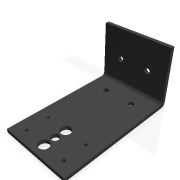
# Autodesk Inventor part: Part5
Saved by Autodesk Inventor 2019 (Build 230136000, 136)
## iProperties
Created: 2019-07-18
Part Number: Part5
Material: Generic
Document SubType Name: Modeling
Designer: romanp
Density: 1 g/cm^3
Appearance: Default
Author: romanp
Autodesk Inventor part; units mm, degrees
ref_plane "YZ Plane" through (0, 0, 0) normal (1, 0, 0) x (0, 1, 0)
ref_plane "XZ Plane" through (0, 0, 0) normal (0, 1, 0) x (-1, 0, 0)
ref_plane "XY Plane" through (0, 0, 0) normal (0, 0, 1) x (1, 0, 0)
sketch "Sketch1" plane through (0, 0, 0) normal (0, 0, 1) x (1, 0, 0)
  line L0 (0, 0) -> (0, 60)
  line L1 (0, 60) -> (70, 60)
  line L2 (70, 60) -> (70, 0)
  line L3 (70, 0) -> (0, 0)
  dimension "d0" = 60
  dimension "d1" = 70
  dimension "d2" = 60
  constraints: 8 end point, 2 perpendicular, 1 vertical
  measures "d0" distance of L0.start L0.end
  measures "d1" distance of L0.end L1.end
  measures "d2" distance of L1.end L2.end
extrude "Extrusion1" add sketch "Sketch1" along normal blind 4
sketch "Sketch2" plane through (0, 0, 4) normal (0, 0, 1) x (1, 0, 0)
  line L0 (0, 0) -> (70, 0) projected
  line L1 (70, 0) -> (70, 60) projected
  line L2 (0, 0) -> (70, 0)
  line L3 (70, 0) -> (70, 4)
  line L4 (70, 4) -> (0, 4)
  line L5 (0, 4) -> (0, 0)
  dimension "d5" = 4
  constraints: 8 end point, 2 parallel, 1 horizontal, 1 perpendicular, 1 point on line
  measures "d5" distance of L3.end L2.end
extrude "Extrusion2" add sketch "Sketch2" along normal blind 115
sketch "Sketch3" plane through (0, 0, 0) normal (0, 0, -1) x (-1, 0, 0)
  line L0 (-70, 60) -> (-70, 0) projected
  circle A0 centre (-50, 30) radius 3
  circle A1 centre (-20, 30) radius 3
  dimension "d15" = 6
  dimension "d16" = 6
  constraints: 2 centre point
  measures "d15" diameter of A0
  measures "d16" diameter of A1
extrude "Extrusion3" cut sketch "Sketch3" against normal blind 10
sketch "Sketch4" plane through (0, 0, 0) normal (0, -1, 0) x (1, 0, 0)
  line L0 (70, 0) -> (70, 119) projected
  line L1 (23, 0) -> (17, 0) projected
  line L2 (17, 0) -> (23, 0)
  circle A0 centre (50, 23) radius 3
  circle A1 centre (20, 23) radius 3
  dimension "d26" = 6
  dimension "d27" = 6
  constraints: 2 centre point, 2 end point, 1 collinear
  measures "d26" diameter of A0
  measures "d27" diameter of A1
extrude "Extrusion4" cut sketch "Sketch4" against normal blind 10
sketch "Sketch5" plane through (0, 0, 0) normal (0, -1, 0) x (1, 0, 0)
  line L0 (70, 4) -> (70, 119) projected
  circle A0 centre (50, 23) radius 3 projected
  circle A1 centre (35, 108.75) radius 5.25
  circle A2 centre (35, 86.75) radius 5.25
  circle A3 centre (35, 97.75) radius 4
  circle A4 centre (55.25, 86.75) radius 2
  circle A5 centre (55.25, 108.75) radius 2
  circle A6 centre (14.75, 86.75) radius 2
  circle A7 centre (14.75, 108.75) radius 2
  point P0 (0, 0)
  point P1 (20, 23)
  dimension "d36" = 8
  dimension "d41" = 4
  dimension "d42" = 4
  dimension "d43" = 4
  dimension "d44" = 4
  constraints: 7 centre point
  measures "d36" diameter of A3
  measures "d41" diameter of A4
  measures "d42" diameter of A5
  measures "d43" diameter of A6
  measures "d44" diameter of A7
extrude "Extrusion5" cut sketch "Sketch5" against normal blind 10 contours A1 | A2 | A3 | A4 | A5 | A6 | A7
sketch "Sketch6" plane through (70, 0, 0) normal (1, 0, 0) x (0, 0, -1)
  line L0 (0, 0) -> (-119, 0) projected
  line L1 (0, 4) -> (0, 4)
  line L2 (-4, 4) -> (-119, 4) projected
  line L3 (0, 60) -> (0, 0) projected
  line L4 (-4, 0) -> (-4, 0)
  arc A0 (-4, 0) -> (0, 4) centre (-4, 4) ccw
  line L5 (0, 4) -> (0, 0)
  line L6 (-4, 0) -> (0, 0)
  dimension "d47" = 4
  dimension "d48" = 4
  dimension "d49" = 4
  constraints: 8 end point, 4 tangent, 3 point on line, 2 collinear, 2 point on circle, 1 centre point, 1 perpendicular
  measures "d47" distance of L0.start L1.end
  measures "d48" distance of L0.start L4.end
  measures "d49" radius of A0
extrude "Extrusion6" cut sketch "Sketch6" against normal blind 100
sketch "Sketch7" plane through (70, 60, 4) normal (1, 0, 0) x (0, 0, -1)
  line L0 (0, -56) -> (0, 0) projected
  line L1 (0, -52) -> (0, -52)
  line L2 (-4, -56) -> (-4, -56)
  arc A0 (-4, -56) -> (0, -52) centre (-4, -52) ccw
  line L3 (0, -52) -> (0, -56)
  line L4 (0, -56) -> (-115, -56) projected
  line L5 (-4, -56) -> (0, -56)
  point P0 (4, -60)
  dimension "d52" = 4
  dimension "d53" = 4
  dimension "d54" = 4
  constraints: 8 end point, 4 tangent, 3 point on line, 2 collinear, 2 point on circle, 1 centre point, 1 horizontal
  measures "d52" distance of L0.start L1.end
  measures "d53" distance of L0.start L2.end
  measures "d54" radius of A0
extrude "Extrusion7" add sketch "Sketch7" against normal blind 70
sketch "Sketch8" plane through (0, 0, 119) normal (0, -1, 0) x (1, 0, 0)
  circle A0 centre (35, -10.25) radius 5.25 projected
  circle A1 centre (55.25, -32.25) radius 2 projected
  circle A2 centre (55.25, -32.25) radius 2
  circle A3 centre (55.25, -10.25) radius 2 projected
  circle A4 centre (55.25, -10.25) radius 2
  circle A5 centre (14.75, -10.25) radius 2 projected
  circle A6 centre (14.75, -10.25) radius 2
  circle A7 centre (14.75, -32.25) radius 2 projected
  circle A8 centre (14.75, -32.25) radius 2
  point P0 (0, -119)
  constraints: 4 centre point, 4 coincident
extrude "Extrusion8" add sketch "Sketch8" against normal blind 4 contours A1 | A3 | A5 | A7
sketch "Sketch9" plane through (0, 0, 119) normal (0, -1, 0) x (1, 0, 0)
  circle A0 centre (35, -10.25) radius 5.25 projected
  circle A1 centre (57.5, -10.25) radius 1.65
  circle A2 centre (12.5, -10.25) radius 1.65
  circle A3 centre (57.5, -32.25) radius 1.65
  circle A4 centre (12.5, -32.25) radius 1.65
  point P0 (0, -119)
  dimension "d62" = 3.3
  dimension "d63" = 3.3
  dimension "d66" = 3.3
  dimension "d67" = 3.3
  constraints: 4 centre point
  measures "d62" diameter of A1
  measures "d63" diameter of A2
  measures "d66" diameter of A3
  measures "d67" diameter of A4
extrude "Extrusion9" cut sketch "Sketch9" against normal blind 4 contours A1 | A2 | A3 | A4
body "Solid1"
